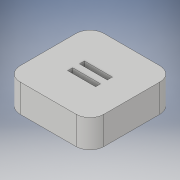
# Autodesk Inventor part: Unit_v2
Saved by Autodesk Inventor 2019 (Build 230136000, 136)
## iProperties
Created: 2018-11-21
Part Number: Unit_v2
Material: Generic
Document SubType Name: Modeling
Designer: Jeffrey Tan
Density: 1 g/cm^3
Appearance: Default
Author: Jeffrey Tan
Autodesk Inventor part; units mm, degrees
ref_plane "YZ Plane" through (0, 0, 0) normal (1, 0, 0) x (0, 1, 0)
ref_plane "XZ Plane" through (0, 0, 0) normal (0, 1, 0) x (-1, 0, 0)
ref_plane "XY Plane" through (0, 0, 0) normal (0, 0, 1) x (1, 0, 0)
sketch "Sketch1" plane through (0, 0, 0) normal (0, 1, 0) x (-1, 0, 0)
  line L0 (-9.525, 9.525) -> (9.525, 9.525)
  line L1 (9.525, 9.525) -> (9.525, -9.525)
  line L2 (9.525, -9.525) -> (-9.525, -9.525)
  line L3 (-9.525, -9.525) -> (-9.525, 9.525)
  point P0 (0, 0)
  dimension "d0" = 19.05
  dimension "d1" = 19.05
  dimension "d2" = 9.525
  dimension "d3" = 9.525
  constraints: 8 end point, 2 parallel, 1 horizontal, 1 perpendicular
  measures "d0" distance of L0.start L0.end
  measures "d1" distance of L0.end L1.end
  measures "d2" distance from line of point (0, 0) L1
  measures "d3" distance from line of L0 point (0, 0)
extrude "Extrusion1" add sketch "Sketch1" along normal blind 6.35
sketch "Sketch2" plane through (0, 6.35, 0) normal (0, 1, 0) x (1, 0, 0)
  line L0 (-3.175, 1.905) -> (3.175, 1.905)
  line L1 (3.175, 1.905) -> (3.175, 0.762)
  line L2 (3.175, 0.762) -> (-3.175, 0.762)
  line L3 (-3.175, 0.762) -> (-3.175, 1.905)
  line L4 (-3.175, -0.762) -> (3.175, -0.762)
  line L5 (3.175, -0.762) -> (3.175, -1.905)
  line L6 (3.175, -1.905) -> (-3.175, -1.905)
  line L7 (-3.175, -1.905) -> (-3.175, -0.762)
  line L8 (0, 1.905) -> (0, 0.762)
  line L9 (0, -1.905) -> (0, -0.762)
  point P0 (0, 0)
  dimension "d6" = 6.35
  dimension "d7" = 1.143
  dimension "d8" = 3.175
  dimension "d11" = 1.524
  dimension "d12" = 0.762
  dimension "d13" = 6.35
  dimension "d14" = 1.143
  constraints: 20 end point, 4 midpoint, 4 parallel, 2 horizontal, 2 perpendicular, 1 collinear
  measures "d6" distance of L1.end L2.end
  measures "d7" distance of L0.end L1.end
  measures "d8" distance from line of point (0, 0) L1
  measures "d11" distance between parallel lines of L4 L2
  measures "d12" distance from line of point (0, 0) L2
  measures "d13" distance between parallel lines of L7 L5
  measures "d14" distance of L4.end L5.end
extrude "Extrusion2" cut sketch "Sketch2" against normal blind 1.143 contours L0 L8 L2 L3 | L4 L9 L6 L7
extrude "Extrusion3" cut sketch "Sketch2" against normal blind 2.286 contours L0 L1 L2 L8 | L4 L5 L6 L9
sketch "Sketch3" plane through (0, 6.35, 0) normal (0, 1, 0) x (1, 0, 0)
  line L0 (0, -0.762) -> (0, -1.905) projected
  circle A0 centre (0, -1.3335) radius 0.5715
  line L1 (0, 0.762) -> (0, 1.905) projected
  circle A1 centre (0, 1.3335) radius 0.5715
  point P0 (0, 0)
  constraints: 2 midpoint, 2 vertical alignment, 4 other
extrude "Extrusion4" cut sketch "Sketch3" against normal through all
fillet "Fillet1" radius 3.175 4 edges at (-9.525, 3.175, 9.525) (9.525, 3.175, 9.525) (9.525, 3.175, -9.525) (-9.525, 3.175, -9.525)
body "Solid1"
